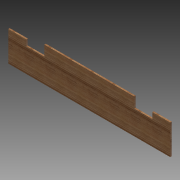
# Autodesk Inventor part: dozer side pannel
Saved by Autodesk Inventor 2012 (Build 160160000, 160)
## iProperties
Created: 2013-10-06
Part Number: dozer side pannel
Material: Default
Document SubType Name: Modeling
Designer: Bryce
Density: 1 g/cm^3
Author: Bryce
Autodesk Inventor part; units mm, degrees
ref_plane "YZ Plane" through (0, 0, 0) normal (1, 0, 0) x (0, 1, 0)
ref_plane "XZ Plane" through (0, 0, 0) normal (0, 1, 0) x (-1, 0, 0)
ref_plane "XY Plane" through (0, 0, 0) normal (0, 0, 1) x (1, 0, 0)
sketch "Sketch1" plane through (0, 0, 0) normal (0, 0, 1) x (1, 0, 0)
  line L0 (0, 0) -> (685.8, 0)
  line L1 (685.8, 0) -> (685.8, 127)
  line L2 (0, 127) -> (0, 0)
  line L3 (152.4, 146.05) -> (152.4, 101.6)
  line L4 (152.4, 101.6) -> (76.2, 101.6)
  line L5 (76.2, 101.6) -> (76.2, 127)
  line L6 (533.4, 146.05) -> (533.4, 101.6)
  line L7 (533.4, 101.6) -> (609.6, 101.6)
  line L8 (609.6, 101.6) -> (609.6, 127)
  line L9 (76.2, 127) -> (0, 127)
  line L10 (685.8, 127) -> (609.6, 127)
  line L11 (533.4, 146.05) -> (152.4, 146.05)
  dimension "d0" = 127
  dimension "d1" = 685.8
  dimension "d4" = 76.2
  dimension "d6" = 76.2
  dimension "d7" = 76.2
  dimension "d8" = 76.2
  dimension "d10" = 25.4
  dimension "d11" = 44.45
  dimension "d12" = 25.4
  constraints: 24 end point, 6 parallel, 3 perpendicular, 1 collinear, 1 horizontal
  measures "d0" distance of L2.start L0.start
  measures "d1" distance of L0.start L0.end
  measures "d4" distance of L3.end L4.end
  measures "d6" distance between parallel lines of L2 L5
  measures "d7" distance between parallel lines of L1 L8
  measures "d8" distance of L6.end L7.end
  measures "d10" distance of L4.end L5.end
  measures "d11" distance of L6.start L6.end
  measures "d12" distance of L7.end L8.end
extrude "Extrusion1" add sketch "Sketch1" along normal blind 6.35
equation "\"d7\" = d6"
equation "\"d8\" = d4"
body "Solid1"
